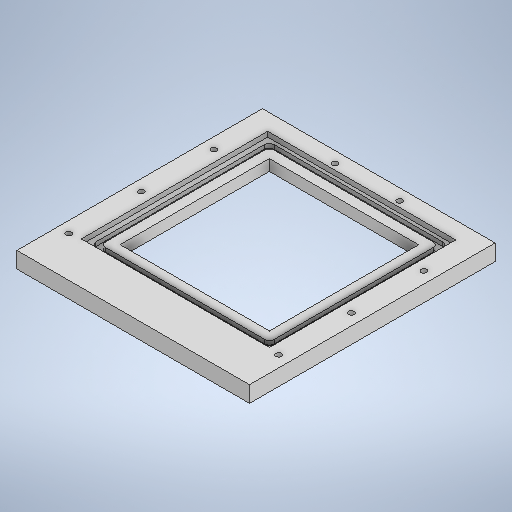
# Autodesk Inventor part: Glass holder
Saved by Autodesk Inventor 2025.2 (Build 292293000, 293)
## iProperties
Created: 2025-08-07
Part Number: Glass holder
Material: Generic
Document SubType Name: Modeling
Designer: mateo
Density: 1 g/cm^3
Appearance: Default
Author: mateo
Autodesk Inventor part; units mm, degrees
ref_plane "YZ Plane" through (0, 0, 0) normal (1, 0, 0) x (0, 1, 0)
ref_plane "XZ Plane" through (0, 0, 0) normal (0, 1, 0) x (-1, 0, 0)
ref_plane "XY Plane" through (0, 0, 0) normal (0, 0, 1) x (1, 0, 0)
sketch "Sketch1" plane through (0, 0, 0) normal (0, 1, 0) x (-1, 0, 0)
  line L0 (72, -76) -> (-72, -76)
  line L1 (-72, -76) -> (-72, 76)
  line L2 (-72, 76) -> (72, 76)
  line L3 (72, 76) -> (72, -76)
  line L4 (72, -76) -> (-72, 76) construction
  line L5 (-72, -76) -> (72, 76) construction
  point P0 (0, 0)
  dimension "d3" = 152
  dimension "d4" = 144
  constraints: 12 end point, 2 midpoint, 2 parallel, 1 horizontal, 1 perpendicular
  measures "d3" distance of L2.end L0.start
  measures "d4" distance of L0.start L0.end
extrude "Extrusion1" add sketch "Sketch1" along normal blind 10
sketch "Sketch2" plane through (0, 10, 0) normal (0, 1, 0) x (1, 0, 0)
  line L0 (-9.5175, -400.0105) -> (-9.5175, -295.6322)
  line L1 (-12.5175, -292.6322) -> (-116.9815, -292.6322)
  line L2 (-119.9815, -295.6322) -> (-119.9815, -400.0105)
  line L3 (-116.9815, -403.0105) -> (-12.5175, -403.0105)
  circle A0 centre (0.2505, -407.097) radius 1.7294
  circle A1 centre (-129.7495, -407.097) radius 1.7294
  circle A2 centre (-84.7495, -287.097) radius 1.7294
  line L4 (-18.5175, -301.6322) -> (-110.9815, -301.6322)
  line L5 (-18.5175, -394.0105) -> (-18.5175, -301.6322)
  line L6 (-110.9815, -301.6322) -> (-110.9815, -394.0105)
  line L7 (-110.9815, -394.0105) -> (-18.5175, -394.0105)
  line L8 (-12.5175, -298.6322) -> (-12.5175, -397.0105)
  line L9 (-15.5175, -400.0105) -> (-113.9815, -400.0105)
  line L10 (-116.9815, -397.0105) -> (-116.9815, -298.6322)
  line L11 (-113.9815, -295.6322) -> (-15.5175, -295.6322)
  arc A3 (-116.9815, -397.0105) -> (-113.9815, -400.0105) centre (-113.9815, -397.0105) ccw
  arc A4 (-119.9815, -400.0105) -> (-116.9815, -403.0105) centre (-116.9815, -400.0105) ccw
  arc A5 (-15.5175, -400.0105) -> (-12.5175, -397.0105) centre (-15.5175, -397.0105) ccw
  arc A6 (-12.5175, -403.0105) -> (-9.5175, -400.0105) centre (-12.5175, -400.0105) ccw
  arc A7 (-9.5175, -295.6322) -> (-12.5175, -292.6322) centre (-12.5175, -295.6322) ccw
  arc A8 (-12.5175, -298.6322) -> (-15.5175, -295.6322) centre (-15.5175, -298.6322) ccw
  arc A9 (-116.9815, -292.6322) -> (-119.9815, -295.6322) centre (-116.9815, -295.6322) ccw
  arc A10 (-113.9815, -295.6322) -> (-116.9815, -298.6322) centre (-113.9815, -298.6322) ccw
  line L12 (-46.232, -37.913) -> (46.232, -37.913)
  line L13 (46.232, -37.913) -> (46.232, 54.465)
  line L14 (46.232, 54.465) -> (-46.232, 54.465)
  line L15 (-46.232, 54.465) -> (-46.232, -37.913)
  line L16 (72, -76) -> (72, 76) construction
  line L17 (72, 76) -> (-72, 76) construction
  point P0 (0, 0)
  point P1 (-67.2495, -360.597)
  dimension "d7" = 9
  dimension "d8" = 9
  dimension "d9" = 9
  dimension "d10" = 9
  dimension "d11" = 3
  dimension "d12" = 3
  dimension "d13" = 92.378
  dimension "d14" = 92.464
  dimension "d15" = 25.768
  dimension "d16" = 21.535
  dimension "d19" = 144
  dimension "d20" = 152
  constraints: 32 end point, 16 point on circle, 16 tangent, 11 centre point, 7 equal radius, 7 perpendicular, 2 parallel, 1 horizontal, 1 vertical, 3 other
  measures "d7" distance between parallel lines of L4 L1
  measures "d8" distance between parallel lines of L0 L5
  measures "d9" distance between parallel lines of L2 L6
  measures "d10" distance between parallel lines of L7 L3
  measures "d11" distance between parallel lines of L0 L8
  measures "d12" radius of A3
  measures "d13" distance of L14.end L12.start
  measures "d14" distance of L12.start L12.end
  measures "d15" distance between parallel lines of L16 L13
  measures "d16" distance between parallel lines of L17 L14
  measures "d19" distance of L16.end L17.end
  measures "d20" distance of L16.start L16.end
extrude "Extrusion2" cut sketch "Sketch2" against normal blind 10 contours L15 L14 L13 L12
sketch "Sketch3" plane through (0, 10, 0) normal (0, 1, 0) x (1, 0, 0)
  line L0 (-46.232, 54.465) -> (46.232, 54.465) construction
  line L1 (72, -76) -> (72, 76) construction
  line L2 (-72, 76) -> (-72, -76) construction
  line L3 (-72, -76) -> (72, -76) construction
  line L4 (72, 76) -> (-72, 76) construction
  point P0 (0, 0)
  point P1 (0, 0)
  point P2 (-65, -6)
  point P3 (-65, 39)
  point P4 (-65, -51)
  point P5 (65, -6)
  point P6 (65, 39)
  point P7 (65, -51)
  point P8 (-20, 69)
  point P9 (20, 69)
  dimension "d21" = 45
  dimension "d22" = 45
  dimension "d23" = 45
  dimension "d24" = 45
  dimension "d25" = 14.535
  dimension "d26" = 14.535
  dimension "d27" = 40
  dimension "d28" = 52
  dimension "d29" = 7
  dimension "d30" = 7
  dimension "d31" = 7
  dimension "d32" = 7
  dimension "d33" = 7
  dimension "d34" = 25
  dimension "d36" = 25
  measures "d21" distance of point (-65, -51) point (-65, -6)
  measures "d22" distance of point (-65, -6) point (-65, 39)
  measures "d23" distance of point (65, -6) point (65, 39)
  measures "d24" distance of point (65, -51) point (65, -6)
  measures "d25" distance from line of L0 point (20, 69)
  measures "d26" distance from line of L0 point (-20, 69)
  measures "d27" distance of point (-20, 69) point (20, 69)
  measures "d28" distance from line of point (20, 69) L1
  measures "d29" distance from line of L2 point (-65, -51)
  measures "d30" distance from line of L2 point (-65, -6)
  measures "d31" distance from line of L1 point (65, -51)
  measures "d32" distance from line of L1 point (65, -6)
  measures "d33" distance from line of L1 point (65, 39)
  measures "d34" distance from line of L3 point (65, -51)
  measures "d36" distance from line of L3 point (-65, -51)
hole "Hole1" at (-65, 10, 6) at (-65, 10, -39) at (-65, 10, 51) at (65, 10, 6) at (65, 10, -39) at (65, 10, 51) at (-20, 10, -69) at (20, 10, -69) direction (0, -1, 0) diameter 3.5 end through all
sketch "Sketch4" plane through (0, 10, 0) normal (0, 1, 0) x (1, 0, 0)
  line L0 (55.232, -43.913) -> (55.232, 60.465)
  line L1 (52.232, 63.465) -> (-52.232, 63.465)
  line L2 (-55.232, 60.465) -> (-55.232, -43.913)
  line L3 (-52.232, -46.913) -> (52.232, -46.913)
  circle A0 centre (502.0315, -140.3134) radius 1.7294
  circle A1 centre (372.0315, -140.3134) radius 1.7294
  circle A2 centre (417.0315, -20.3134) radius 1.7294
  line L4 (46.232, 54.465) -> (-46.232, 54.465)
  line L5 (46.232, -37.913) -> (46.232, 54.465)
  line L6 (-46.232, 54.465) -> (-46.232, -37.913)
  line L7 (-46.232, -37.913) -> (46.232, -37.913)
  line L8 (52.232, 57.465) -> (52.232, -40.913)
  line L9 (49.232, -43.913) -> (-49.232, -43.913)
  line L10 (-52.232, -40.913) -> (-52.232, 57.465)
  line L11 (-49.232, 60.465) -> (49.232, 60.465)
  arc A3 (-52.232, -40.913) -> (-49.232, -43.913) centre (-49.232, -40.913) ccw
  arc A4 (-55.232, -43.913) -> (-52.232, -46.913) centre (-52.232, -43.913) ccw
  arc A5 (49.232, -43.913) -> (52.232, -40.913) centre (49.232, -40.913) ccw
  arc A6 (52.232, -46.913) -> (55.232, -43.913) centre (52.232, -43.913) ccw
  arc A7 (55.232, 60.465) -> (52.232, 63.465) centre (52.232, 60.465) ccw
  arc A8 (52.232, 57.465) -> (49.232, 60.465) centre (49.232, 57.465) ccw
  arc A9 (-52.232, 63.465) -> (-55.232, 60.465) centre (-52.232, 60.465) ccw
  arc A10 (-49.232, 60.465) -> (-52.232, 57.465) centre (-49.232, 57.465) ccw
  line L12 (-46.232, 54.465) -> (46.232, 54.465) projected
  line L13 (46.232, -37.913) -> (-46.232, -37.913) projected
  line L14 (46.232, 54.465) -> (46.232, -37.913) projected
  line L15 (-46.232, -37.913) -> (-46.232, 54.465) projected
  point P0 (0, 0)
  point P1 (-14.6695, 0.7102)
  dimension "d44" = 9
  dimension "d45" = 9
  dimension "d46" = 9
  dimension "d47" = 9
  dimension "d48" = 3
  dimension "d49" = 3
  dimension "d51" = 0
  dimension "d52" = 0
  dimension "d53" = 0
  dimension "d54" = 0
  constraints: 22 end point, 16 point on circle, 16 tangent, 11 centre point, 7 equal radius, 6 perpendicular, 1 horizontal alignment, 1 vertical, 5 other
  measures "d45" distance between parallel lines of L0 L5
  measures "d46" distance between parallel lines of L2 L6
  measures "d47" distance between parallel lines of L7 L3
  measures "d48" distance between parallel lines of L0 L8
  measures "d49" radius of A3
  measures "d51" vertical extent of L12
  measures "d52" distance between parallel lines of L13 L7
  measures "d53" distance between parallel lines of L14 L5
  measures "d54" distance between parallel lines of L15 L6
extrude "Extrusion3" cut sketch "Sketch4" against normal blind 2.5 contours A6 L3 A4 L2 A9 L1 A7 L0
sketch "Sketch5" plane through (0, 10, 0) normal (0, 1, 0) x (1, 0, 0)
  line L0 (58.232, -49.913) -> (-58.232, -49.913)
  line L1 (-58.232, -49.913) -> (-58.232, 65.465)
  line L2 (-58.232, 65.465) -> (58.232, 65.465)
  line L3 (58.232, 65.465) -> (58.232, -49.913)
  line L4 (72, 76) -> (-72, 76) projected
  line L5 (-55.232, -43.913) -> (-55.232, 60.465) projected
  line L6 (55.232, 60.465) -> (55.232, -43.913) projected
  line L7 (52.232, -46.913) -> (-52.232, -46.913) projected
  line L8 (-52.232, 63.465) -> (52.232, 63.465) projected
  point P0 (0, 0)
  point P1 (58.232, 76)
  point P2 (-58.232, 76)
  dimension "d58" = 3
  dimension "d59" = 3
  dimension "d60" = 3
  dimension "d65" = 2
  constraints: 8 end point, 2 parallel, 1 horizontal, 1 perpendicular
  measures "d58" distance between parallel lines of L1 L5
  measures "d59" distance between parallel lines of L6 L3
  measures "d60" distance between parallel lines of L7 L0
  measures "d65" distance between parallel lines of L2 L8
extrude "Extrusion4" cut sketch "Sketch5" against normal blind 3.1
extrude "Extrusion5" cut sketch "Sketch4" against normal blind 5.6 contours A6 L3 A4 L2 A9 L1 A7 L0
body "Solid1"
